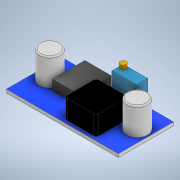
# Autodesk Inventor part: Control and Power Box
Saved by Autodesk Inventor 2022 (Build 260153000, 153)
## iProperties
Created: 2021-10-17
Part Number: Control and Power Box
Material: Generic
Document SubType Name: Modeling
Designer: dech3
Density: 1 g/cm^3
Appearance: Default
Author: dech3
Autodesk Inventor part; units mm, degrees
ref_plane "YZ Plane" through (0, 0, 0) normal (1, 0, 0) x (0, 1, 0)
ref_plane "XZ Plane" through (0, 0, 0) normal (0, 1, 0) x (-1, 0, 0)
ref_plane "XY Plane" through (0, 0, 0) normal (0, 0, 1) x (1, 0, 0)
sketch "Sketch1" plane through (0, 0, 0) normal (0, 1, 0) x (-1, 0, 0)
  line L0 (21.5, -10.6) -> (-21.5, -10.6)
  line L1 (-21.5, -10.6) -> (-21.5, 10.6)
  line L2 (-21.5, 10.6) -> (21.5, 10.6)
  line L3 (21.5, 10.6) -> (21.5, -10.6)
  point P0 (0, 0)
  dimension "d0" = 43
  dimension "d1" = 21.2
  dimension "d2" = 10.6
  dimension "d3" = 21.5
  constraints: 8 end point, 2 parallel, 1 horizontal, 1 perpendicular
  measures "d0" distance between parallel lines of L1 L3
  measures "d1" distance between parallel lines of L2 L0
  measures "d2" distance from line of point (0, 0) L0
  measures "d3" distance from line of point (0, 0) L1
extrude "Extrusion1" add sketch "Sketch1" along normal blind 1.31
sketch "Sketch2" plane through (0, 1.31, 0) normal (0, 1, 0) x (1, 0, 0)
  line L0 (-12, 10) -> (-1.85, 10)
  line L1 (-1.85, 10) -> (-1.85, -2.4)
  line L2 (-1.85, -2.4) -> (-12, -2.4)
  line L3 (-12, -2.4) -> (-12, 10)
  line L4 (-21.5, -10.6) -> (21.5, -10.6) projected
  line L5 (-21.5, 10.6) -> (-21.5, -10.6) projected
  point P0 (0, 0)
  dimension "d6" = 12.4
  dimension "d7" = 10.15
  dimension "d8" = 8.2
  dimension "d9" = 9.5
  constraints: 8 end point, 2 parallel, 1 horizontal, 1 perpendicular
  measures "d6" distance between parallel lines of L2 L0
  measures "d7" distance between parallel lines of L1 L3
  measures "d8" distance between parallel lines of L4 L2
  measures "d9" distance between parallel lines of L5 L3
extrude "Extrusion2" add sketch "Sketch2" along normal blind 4
sketch "Sketch3" plane through (0, 1.31, 0) normal (0, 1, 0) x (1, 0, 0)
  line L0 (0.6, 2.8) -> (10.8, 2.8)
  line L1 (11.8, 1.8) -> (11.8, -8.4)
  line L2 (10.8, -9.4) -> (0.6, -9.4)
  line L3 (-0.4, -8.4) -> (-0.4, 1.8)
  line L4 (-21.5, -10.6) -> (21.5, -10.6) projected
  line L5 (21.5, -10.6) -> (21.5, 10.6) projected
  arc A0 (0.6, 2.8) -> (-0.4, 1.8) centre (0.6, 1.8) ccw
  arc A1 (11.8, 1.8) -> (10.8, 2.8) centre (10.8, 1.8) ccw
  arc A2 (10.8, -9.4) -> (11.8, -8.4) centre (10.8, -8.4) ccw
  arc A3 (-0.4, -8.4) -> (0.6, -9.4) centre (0.6, -8.4) ccw
  point P0 (0, 0)
  dimension "d12" = 12.2
  dimension "d13" = 12.2
  dimension "d14" = 1.2
  dimension "d15" = 9.7
  dimension "d16" = 1
  constraints: 8 end point, 8 point on circle, 8 tangent, 4 centre point, 3 equal radius, 2 parallel, 1 horizontal, 1 perpendicular
  measures "d12" distance between parallel lines of L2 L0
  measures "d13" distance between parallel lines of L1 L3
  measures "d14" distance between parallel lines of L4 L2
  measures "d15" distance between parallel lines of L5 L1
  measures "d16" radius of A0
extrude "Extrusion3" add sketch "Sketch3" along normal blind 7.4
sketch "Sketch4" plane through (0, 1.31, 0) normal (0, 1, 0) x (1, 0, 0)
  line L0 (2.66, 10.1) -> (12.13, 10.1)
  line L1 (12.13, 10.1) -> (12.13, 5.79)
  line L2 (12.13, 5.79) -> (2.66, 5.79)
  line L3 (2.66, 5.79) -> (2.66, 10.1)
  line L4 (21.5, -10.6) -> (21.5, 10.6) projected
  line L5 (21.5, 10.6) -> (-21.5, 10.6) projected
  point P0 (0, 0)
  dimension "d19" = 4.31
  dimension "d20" = 9.47
  dimension "d21" = 9.37
  dimension "d22" = 0.5
  constraints: 8 end point, 2 parallel, 1 horizontal, 1 perpendicular
  measures "d19" distance between parallel lines of L2 L0
  measures "d20" distance between parallel lines of L1 L3
  measures "d21" distance between parallel lines of L1 L4
  measures "d22" distance between parallel lines of L5 L0
extrude "Extrusion4" add sketch "Sketch4" along normal blind 10
sketch "Sketch5" plane through (0, 11.31, 0) normal (0, 1, 0) x (1, 0, 0)
  circle A0 centre (3.86, 8.9) radius 1.125
  line L0 (12.13, 10.1) -> (2.66, 10.1) projected
  line L1 (2.66, 10.1) -> (2.66, 5.79) projected
  point P0 (0, 0)
  point P1 (2.66, 9.2358)
  point P2 (2.66, 8.7642)
  point P3 (4.0958, 10.1)
  point P4 (3.6242, 10.1)
  dimension "d25" = 2.25
  dimension "d26" = 1.2
  dimension "d27" = 1.2
  constraints: 1 centre point
  measures "d25" diameter of A0
  measures "d26" distance from line of L0 A0.centre
  measures "d27" distance from line of L1 A0.centre
extrude "Extrusion5" add sketch "Sketch5" along normal blind 1.61
sketch "Sketch6" plane through (0, 1.31, 0) normal (0, 1, 0) x (1, 0, 0)
  circle A0 centre (-16.28, 0.87) radius 4
  circle A1 centre (16.93, 1.23) radius 4
  line L0 (-21.5, -10.6) -> (21.5, -10.6) projected
  line L1 (21.5, -10.6) -> (21.5, 10.6) projected
  line L2 (-21.5, 10.6) -> (-21.5, -10.6) projected
  point P0 (0, 0)
  dimension "d30" = 8
  dimension "d31" = 8
  dimension "d32" = 11.83
  dimension "d33" = 4.57
  dimension "d34" = 5.22
  dimension "d35" = 11.47
  constraints: 2 centre point
  measures "d30" diameter of A0
  measures "d31" diameter of A1
  measures "d32" distance from line of L0 A1.centre
  measures "d33" distance from line of L1 A1.centre
  measures "d34" distance from line of L2 A0.centre
  measures "d35" distance from line of L0 A0.centre
extrude "Extrusion6" add sketch "Sketch6" along normal blind 10.5
fillet "Fillet1" radius 0.5 2 edges at (12.93, 11.81, -1.23) (-20.28, 11.81, -0.87)
equation "\"d2\" = 0.5 * d1"
equation "\"d3\" = 0.5 * d0"
body "Solid1"
